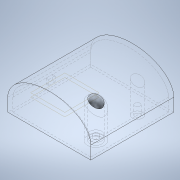
# Autodesk Inventor part: base_snap_test
Saved by Autodesk Inventor 2021 (Build 250183000, 183)
## iProperties
Created: 2023-08-20
Part Number: base_snap_test
Material: Genérico
Document SubType Name: Modeling
Designer: Sergio
Density: 1 g/cm^3
Appearance: Valor por defecto
Author: Sergio
Autodesk Inventor part; units mm, degrees
ref_plane "YZ Plane" through (0, 0, 0) normal (1, 0, 0) x (0, 1, 0)
ref_plane "XZ Plane" through (0, 0, 0) normal (0, 1, 0) x (-1, 0, 0)
ref_plane "XY Plane" through (0, 0, 0) normal (0, 0, 1) x (1, 0, 0)
sketch "Boceto1" plane through (0, 0, 0) normal (0, 0, 1) x (1, 0, 0)
  line L0 (0, 4) -> (-2, 4)
  line L1 (0, 0) -> (2.5, 0)
  line L2 (2.5, 4) -> (2.5, 7)
  line L3 (2.5, 7) -> (0, 7)
  line L4 (0, 7) -> (-2, 5)
  line L5 (0, -5.5) -> (0, 0)
  line L6 (2.5, 4) -> (2.5, 0)
  line L7 (2.5, 0) -> (2.5, -2.1716)
  line L8 (1.9142, -3.5858) -> (1.1716, -4.3284)
  line L9 (0, 4) -> (0.25, 4)
  line L10 (0.25, 4) -> (0.25, 0)
  line L11 (-2, 4) -> (-2, 5)
  arc A0 (1.9142, -3.5858) -> (2.5, -2.1716) centre (0.5, -2.1716) ccw
  line L12 (0, -7.1569) -> (0, -10.5)
  arc A1 (1.1716, -4.3284) -> (0, -7.1569) centre (4, -7.1569) ccw
  point P0 (2.5, -3)
  dimension "d0" = 2.5
  dimension "d2" = 3
  dimension "d3" = 4
  dimension "d4" = 4
  dimension "d27" = 0.25
  dimension "d28" = 45
  dimension "d29" = 2
  dimension "d30" = 1
  dimension "d31" = 3
  dimension "d32" = 45
  dimension "d33" = 2
  dimension "d34" = 5
  dimension "d35" = 4
  constraints: 26 end point, 6 point on line, 4 point on circle, 4 tangent, 4 vertical, 2 centre point, 2 horizontal, 2 perpendicular
  measures "d0" distance of L1.start L1.end
  measures "d2" distance of L2.start L2.end
  measures "d3" distance of L1.start L0.start
  measures "d4" distance of L1.end L2.start
  measures "d27" distance of L0.start L9.end
  measures "d28" angle of L0 L4
  measures "d29" distance of L0.start L0.end
  measures "d30" distance of L0.end L4.end
  measures "d31" distance of L1.end point (2.5, -3)
  measures "d32" angle of L5 L8
  measures "d33" radius of A0
  measures "d34" distance of L5.start L12.end
  measures "d35" radius of A1
sketch "Boceto2" plane through (0, 0, 0) normal (0, 1, 0) x (-1, 0, 0)
  line L0 (0, 0) -> (2, 0)
  line L1 (0, 0) -> (-30, 0)
  line L2 (-62, -32) -> (2, -32)
  line L3 (2, -32) -> (2, 32)
  line L4 (2, 32) -> (-62, 32)
  line L5 (-62, 32) -> (-62, -32)
  line L6 (-62, -32) -> (2, 32) construction
  line L7 (2, -32) -> (-62, 32) construction
  dimension "d6" = 2
  dimension "d7" = 30
  dimension "d8" = 64
  dimension "d9" = 64
  constraints: 16 end point, 3 horizontal, 2 midpoint, 2 parallel, 1 perpendicular
  measures "d6" distance of L0.start L0.end
  measures "d7" distance of L0.start L1.end
  measures "d8" distance of L4.end L3.end
  measures "d9" distance of L3.end L2.end
extrude "Extrusión1" add sketch "Boceto2" along normal blind 40 and the other way blind 20
shell "Vaciado1" thickness 2 removed faces 0
ref_plane "Plano de trabajo2" through (0, 0, 0) normal (0, -1, 0) x (1, 0, 0)
sketch "Boceto3" plane through (0, 0, 0) normal (0, -1, 0) x (1, 0, 0)
  line L0 (60, 30) -> (60, -30) projected
  line L1 (60, 0) -> (50, 0)
  line L2 (50, 0) -> (50, -16)
  line L3 (50, 0) -> (50, 16)
  circle A0 centre (50, -16) radius 4
  circle A1 centre (50, 16) radius 6.5
  point P0 (0, 0)
  dimension "d20" = 10
  dimension "d21" = 16
  dimension "d22" = 16
  dimension "d23" = 8
  dimension "d24" = 13
  constraints: 6 end point, 2 centre point, 2 coincident, 2 vertical, 1 horizontal, 1 midpoint
  measures "d20" distance of L1.start L1.end
  measures "d21" distance of L1.end L2.end
  measures "d22" distance of L1.end L3.end
  measures "d23" diameter of A0
  measures "d24" diameter of A1
extrude "Extrusión2" add sketch "Boceto3" against normal through all
sketch "Boceto4" plane through (0, 0, 0) normal (0, -1, 0) x (1, 0, 0)
  line L0 (81.7327, 42.0826) -> (-20.271, 42.0826)
  line L1 (-20.271, 42.0826) -> (-20.271, -44.6773)
  line L2 (-20.271, -44.6773) -> (81.7327, -44.6773)
  line L3 (81.7327, -44.6773) -> (81.7327, 42.0826)
  point P0 (0, 0)
  constraints: 8 end point, 2 parallel, 1 horizontal, 1 perpendicular
extrude "Extrusión3" cut sketch "Boceto4" along normal through all
sketch "Boceto11" plane through (0, 0, 0) normal (0, 0, 1) x (1, 0, 0)
  line L0 (0, 38) -> (0, 0) projected
  line L1 (0, 0) -> (0, 10)
  line L2 (62, 0) -> (62, 40) projected
  line L3 (-2, 0) -> (-2, 40) projected
  line L4 (0, 10) -> (-2, 10)
  line L5 (-2, 10) -> (62, 10)
  ellipse E0 centre (30, 10) end of major axis (-2, 10) minor radius 20 (62, 10) -> (-2, 10) ccw
  line L6 (92, 10) -> (-32, 10)
  spline S0 degree 5 poles (92, 10) (92, 10.5338) (91.9916, 11.0676) (91.9748, 11.6012) (91.6448, 18.6003) (89.8774, 25.5098) (87.0392, 31.4975) (80.0102, 41.3589) (70.4895, 48.7829) (65.7385, 51.6302) (55.9882, 56.1491) (45.5655, 58.7497) (40.4069, 59.5833) (30, 60.4167) (19.5931, 59.5833) (14.4345, 58.7497) (4.0118, 56.1491) (-5.7385, 51.6302) (-10.4895, 48.7829) (-20.0102, 41.3589) (-27.0392, 31.4975) (-29.8774, 25.5098) (-31.6448, 18.6003) (-31.9748, 11.6012) (-31.9916, 11.0676) (-32, 10.5338) (-32, 10) knots 0 0 0 0 0 0 0.015077 0.015077 0.015077 0.197876 0.197876 0.197876 0.353026 0.353026 0.353026 0.5 0.5 0.5 0.646974 0.646974 0.646974 0.802124 0.802124 0.802124 0.984923 0.984923 0.984923 1 1 1 1 1 1
  dimension "d95" = 20
  dimension "d96" = 30
  dimension "d69" = 10
  constraints: 8 end point, 5 point on line, 2 horizontal, 1 midpoint, 1 perpendicular, 9 other
  measures "d69" distance of L0.end L1.end
sketch "Boceto12" plane through (0, 0, 0) normal (0, 0, 1) x (1, 0, 0)
  line L0 (0, 18) -> (0, 0)
  line L1 (0, 0) -> (0, 10)
  line L2 (62, 0) -> (62, 20)
  line L3 (0, 10) -> (-2, 10)
  line L4 (-2, 0) -> (-2, 20)
  line L5 (-2, 10) -> (62, 10)
  ellipse E0 centre (30, 10) end of major axis (-2, 10) minor radius 20 (62, 10) -> (-2, 10) ccw
  line L6 (-2, 10) -> (62, 10)
  line L7 (62, 0) -> (62, 40) projected
  spline S0 degree 5 poles (60.0001, 10) (60.0001, 11.2143) (59.8243, 12.4281) (59.4731, 13.6074) (58.264, 16.3537) (56.3653, 18.7043) (55.0833, 19.9412) (51.9622, 22.4183) (48.4287, 24.2735) (46.3967, 25.1367) (41.973, 26.6492) (37.3809, 27.537) (34.9292, 27.8456) (30, 28.1544) (25.0708, 27.8456) (22.6191, 27.537) (18.027, 26.6492) (13.6033, 25.1367) (11.5713, 24.2735) (8.0378, 22.4183) (4.9167, 19.9412) (3.6347, 18.7043) (1.736, 16.3537) (0.5269, 13.6074) (0.1757, 12.4281) (-0.0001, 11.2143) (-0.0001, 10) knots 0 0 0 0 0 0 0.079367 0.079367 0.079367 0.195066 0.195066 0.195066 0.338891 0.338891 0.338891 0.5 0.5 0.5 0.661109 0.661109 0.661109 0.804934 0.804934 0.804934 0.920633 0.920633 0.920633 1 1 1 1 1 1
  point P0 (0, 16.9597)
  dimension "d76" = 20
  dimension "d97" = 2
  dimension "d70" = 10
  constraints: 14 end point, 3 midpoint, 2 point on line, 1 horizontal, 1 perpendicular, 7 other
  measures "d70" distance of L0.end L1.end
extrude "Extrusión9" cut sketch "Boceto11" along normal through all both and the other way through all contours E0 L6 S0
extrude "Extrusión10" add sketch "Boceto12" along normal mid plane 64 contours E0 L5 S0 L0
sketch "Boceto5" plane through (50, 0, -16) normal (0, -1, 0) x (1, 0, 0)
  circle A0 centre (0, 0) radius 4 projected
  circle A1 centre (0, 0) radius 2
  point P0 (-50, 16)
  dimension "d38" = 4
  constraints: 1 centre point, 1 coincident
  measures "d38" diameter of A1
extrude "Extrusión4" cut sketch "Boceto5" against normal blind 7 contours A1
sketch "Boceto6" plane through (50, 0, 16) normal (0, -1, 0) x (1, 0, 0)
  circle A0 centre (0, 0) radius 2
  point P0 (-50, -16)
  dimension "d42" = 4
  constraints: 1 centre point
  measures "d42" diameter of A0
hole "Agujero1" at (50, 0, 16) direction (0, 1, 0) diameter 4 depth 10
ref_plane "Plano de trabajo3" through (0, 3, 0) normal (0, -1, 0) x (1, 0, 0)
sketch "Boceto8" plane through (0, 3, 0) normal (0, -1, 0) x (1, 0, 0)
  line L0 (0, 0) -> (50, 0)
  circle A0 centre (50, 16) radius 2 projected
  line L1 (50, 0) -> (50, 16)
  circle A1 centre (50, 16) radius 4.5
  dimension "d56" = 50
  dimension "d57" = 9
  constraints: 4 end point, 1 centre point, 1 coincident, 1 horizontal
  measures "d56" distance of L0.start L0.end
  measures "d57" diameter of A1
extrude "Extrusión6" cut sketch "Boceto8" against normal through all contours A0 | A1
sketch "Boceto10" plane through (-2, 40, -32) normal (-1, 0, 0) x (0, 0, 1)
  line L0 (32, -40) -> (32, -36)
  line L1 (32, -36) -> (29.5, -36)
  line L2 (29.5, -36) -> (29.5, -32)
  line L3 (29.5, -32) -> (34.5, -32)
  line L4 (34.5, -32) -> (34.5, -36)
  line L5 (34.5, -36) -> (32, -36)
  dimension "d63" = 4
  dimension "d64" = 2.5
  dimension "d65" = 4
  dimension "d66" = 5
  constraints: 12 end point, 5 perpendicular, 1 point on line, 1 vertical
  measures "d63" distance of L0.start L0.end
  measures "d64" distance of L0.end L1.end
  measures "d65" distance of L1.end L2.end
  measures "d66" distance of L2.end L3.end
extrude "Extrusión8" cut sketch "Boceto10" against normal up to surface (2 mm away)
thread "Rosca1" size "M4x0.7" class "6H" standard "ANSI Metric M Profile" full length
sketch "Boceto15" plane through (50, 0, 16) normal (0, -1, 0) x (1, 0, 0)
  circle A0 centre (0, 0) radius 2 projected
  circle A1 centre (0, 0) radius 6.5
  point P0 (-50, -16)
  dimension "d87" = 13
  constraints: 1 centre point, 1 coincident
  measures "d87" diameter of A1
extrude "Extrusión13" cut sketch "Boceto15" against normal blind 1
sketch "Boceto16" plane through (50, 1, 16) normal (0, -1, 0) x (1, 0, 0)
  circle A0 centre (0, 0) radius 6.5
  circle A1 centre (0, 0) radius 2 projected
  circle A2 centre (0, 0) radius 4.5
  point P0 (-50, -16)
  dimension "d90" = 13
  dimension "d91" = 9
  constraints: 2 centre point, 1 coincident
  measures "d90" diameter of A0
  measures "d91" diameter of A2
extrude "Extrusión14" add sketch "Boceto16" along normal blind 2 contours A0
equation "\"d0\" = sf_head_width - sf_head_grip_width"
equation "\"d2\" = sf_head_height"
equation "\"d3\" = d4"
equation "\"d4\" = sf_lenght - sf_head_height"
equation "\"d27\" = sf_head_offset"
equation "\"d28\" = sf_head_angle"
equation "\"d29\" = sf_head_grip_width"
equation "\"d31\" = sf_base"
equation "\"d8\" = 2 * d6 + 2 * d7"
equation "\"d9\" = 2 * d6 + 2 * d7"
equation "\"d21\" = 0.25 * d9"
equation "\"d22\" = 0.25 * d9"
equation "\"d23\" = gj_D"
equation "\"d24\" = screwJ_top_D"
equation "\"d97\" = thikness"
equation "\"d38\" = gj_d"
equation "\"d39\" = gj_out_section + offset"
equation "\"d42\" = screw_d"
equation "\"d48\" = screw_lenght - thikness"
equation "\"d57\" = screw_Dhead + offset"
equation "\"d63\" = sf_lenght - sf_head_height"
equation "\"d64\" = 0.5 * sf_thikness"
equation "\"d65\" = sf_head_height + offset"
equation "\"d66\" = sf_thikness"
equation "\"d87\" = screwJ_top_D"
equation "\"d88\" = 0.5 * thikness"
equation "\"d90\" = screwJ_top_D"
equation "\"d91\" = screwJ_base_D"
equation "\"d92\" = thikness"
equation "\"sf_lenght\" = 7"
equation "\"sf_base\" = 3"
equation "\"sf_head_height\" = 3"
equation "\"sf_head_offset\" = 0.25"
equation "\"sf_head_angle\" = 45deg"
equation "\"sf_head_width\" = 4.5"
equation "\"sf_head_grip_width\" = 2"
equation "\"thikness\" = 2"
equation "\"offset\" = 1"
equation "\"r1\" = 3.5"
equation "\"r2o\" = 60.25"
equation "\"delta_y\" = 6"
equation "\"wire_d\" = 1"
equation "\"width_ang_spring\" = 5"
equation "\"spring_int_diam\" = 8.5"
equation "\"spring_ext_diam\" = 10.5"
equation "\"r3\" = 8.25"
equation "\"r3R\" = 4.75"
equation "\"r3T\" = 6.74537"
equation "\"alpha\" = 54.847297deg"
equation "\"alpha2\" = 270deg"
equation "\"theta3_recogido\" = 305.152703deg"
equation "\"delta_theta_3\" = 45deg"
equation "\"joint_width\" = 12"
equation "\"joint_radius\" = 7.75"
equation "\"shaft_width\" = 15"
equation "\"shaft_joint_diameter\" = 3.875"
equation "\"separation_space\" = 0.5"
equation "\"height_finger\" = 42"
equation "\"cell_screw_head_diameter\" = 4"
equation "\"cell_screw_diameter\" = 2"
equation "\"cell_space\" = 2"
equation "\"cell_width\" = 6"
equation "\"cell_theta_position\" = 60deg"
equation "\"cell_thikness\" = 1"
equation "\"cell_lenght\" = 37"
equation "\"cell_z_space\" = 5"
equation "\"wire_D\" = 3.5"
equation "\"width_link\" = 8"
equation "\"Dt\" = 1.05972"
equation "\"Djoint_shaft\" = 4"
equation "\"shaft_x\" = -0.44028"
equation "\"shaft_y\" = 6.5"
equation "\"lenght_body_link\" = 185.5"
equation "\"lenght_bar_support\" = 202"
equation "\"trigger_offset\" = 2"
equation "\"m2_theta2o\" = 107deg"
equation "\"m2_r2\" = 28"
equation "\"e\" = 9"
equation "\"So\" = 17"
equation "\"m2_theta3o\" = -30deg"
equation "\"m2_r3\" = 19.75"
equation "\"m2_delta_theta1\" = 15deg"
equation "\"m2_theta3f\" = -60deg"
equation "\"trigger_thumb_lenght\" = 6"
equation "\"width_r12\" = 8"
equation "\"m2_r1\" = 25.2"
equation "\"r3_thikness\" = 3.5"
equation "\"t_thikness\" = 3"
equation "\"tg_width\" = 4"
equation "\"pivot_screw_d\" = 4"
equation "\"pivot_diameter\" = 7"
equation "\"sj_diam_shaft\" = 6"
equation "\"sj_groove\" = 2"
equation "\"sj_groove_deep\" = 7"
equation "\"sj_head_D\" = 7"
equation "\"sj_head_d\" = 4.7464"
equation "\"sj_head_height\" = 5"
equation "\"sf_thikness\" = 5"
equation "\"screw_Dhead\" = 8"
equation "\"screw_d\" = 4"
equation "\"screw_lenght\" = 12"
equation "\"screwJ_base_D\" = 9"
equation "\"screwJ_top_D\" = 13"
equation "\"gj_D\" = 8"
equation "\"gj_d\" = 4"
equation "\"gj_out_section\" = 6"
equation "\"d55\" = -1.5 * thikness"
